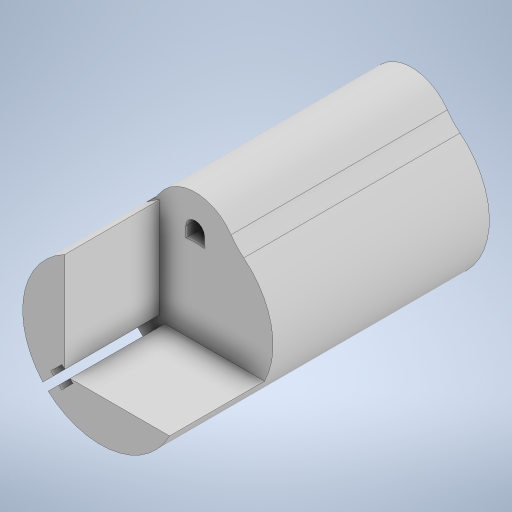
# Autodesk Inventor part: LandingFoot2
Saved by Autodesk Inventor 2023 (Build 270158000, 158)
## iProperties
Created: 2023-01-25
Part Number: LandingFoot2
Material: Generic
Document SubType Name: Modeling
Designer: chase
Density: 1 g/cm^3
Appearance: Default
Author: chase
Autodesk Inventor part; units mm, degrees
ref_plane "YZ Plane" through (0, 0, 0) normal (1, 0, 0) x (0, 1, 0)
ref_plane "XZ Plane" through (0, 0, 0) normal (0, 1, 0) x (-1, 0, 0)
ref_plane "XY Plane" through (0, 0, 0) normal (0, 0, 1) x (1, 0, 0)
sketch "Sketch1" plane through (0, 0, 0) normal (0, 0, 1) x (1, 0, 0)
  circle A0 centre (0, 0) radius 12.5
  dimension "d0" = 25
  constraints: 1 centre point, 1 coincident
  measures "d0" diameter of A0
extrude "Extrusion1" add sketch "Sketch1" against normal blind 50
sketch "Sketch2" plane through (0, 0, -50) normal (0, 0, -1) x (-1, 0, 0)
  circle A0 centre (0, 0) radius 8.075
  dimension "d3" = 16.15
  constraints: 1 centre point, 1 coincident
  measures "d3" diameter of A0
extrude "Extrusion2" cut sketch "Sketch2" against normal blind 25.4
sketch "Sketch3" plane through (0, 0, 0) normal (0, 0, 1) x (1, 0, 0)
  circle A0 centre (0, 0) radius 12.5
  line L0 (0, 12.5) -> (0, 0) construction
  line L1 (0, 0) -> (-8.8388, -8.8388) construction
  line L2 (-4.4194, -2.6517) -> (-9.7227, -7.955)
  line L3 (-9.7227, -7.955) -> (-7.955, -9.7227)
  line L4 (-7.955, -9.7227) -> (-2.6517, -4.4194)
  line L5 (-9.7227, -7.955) -> (-7.955, -9.7227)
  line L6 (-6.1872, -4.4194) -> (-4.4194, -6.1872)
  line L7 (-7.955, -6.1872) -> (-6.1872, -7.955)
  line L8 (-8.4146, -9.2631) -> (-6.6468, -7.4953)
  line L9 (-9.2631, -8.4146) -> (-7.4953, -6.6468)
  line L10 (-4.4194, -2.6517) -> (-2.6517, -4.4194)
  line L11 (-4.879, -5.7276) -> (-4.5255, -5.374)
  line L12 (-5.7276, -4.879) -> (-5.374, -4.5255)
  line L13 (-5.374, -4.5255) -> (-4.5255, -5.374)
  line L14 (-4.9497, -4.9497) -> (-3.5355, -3.5355)
  line L15 (-5.2679, -4.6315) -> (-3.8537, -3.2173)
  line L16 (-4.6315, -5.2679) -> (-3.2173, -3.8537)
  line L17 (-4.4194, -2.6517) -> (-2.6517, -4.4194)
  line L18 (-4.879, -5.7276) -> (11.1106, -5.7276)
  line L19 (-5.7276, -4.879) -> (-5.7276, 11.1106)
  constraints: 40 end point, 6 point on line, 1 vertical, 3 other
extrude "Extrusion3" cut sketch "Sketch3" against normal blind 15.24 contours A0 L18 L4 L10 L2 L19 | L2 L10 L15 L13 L12 L19 | L18 L11 L13 L16 L10 L4 | L9 L7 L8 A0 | A0 L3 L9 | L2 L6 L4 L7 | L12 L13 L11 L6 | L8 L3 A0 | L10 L14 L13 L15 | L16 L13 L14 L10
sketch "Sketch4" plane through (0, 0, -50) normal (0, 0, -1) x (-1, 0, 0)
  arc A0 (6.4283, 10.7204) -> (-6.4283, 10.7204) centre (0, 8.075) ccw
  arc A1 (1.5, 7.9345) -> (-1.5, 7.9345) centre (0, 0) ccw
  circle A2 centre (0, 0) radius 12.5
  point P0 (0, 8.075)
  dimension "d17" = 12.8567
  dimension "d18" = 6.4283
  constraints: 8 point on circle, 3 centre point
  measures "d17" distance of A0.start A0.end
  measures "d18" horizontal distance of A0.start point (0, 8.075)
extrude "Extrusion4" add sketch "Sketch4" against normal up to surface (34.76 mm away) contours A2 A0
sketch "Sketch5" plane through (0, 0, -50) normal (0, 0, -1) x (-1, 0, 0)
  circle A0 centre (0, 9.575) radius 1.5
  line L0 (-1.5, 9.575) -> (-1.5, 7.9345)
  line L1 (1.5, 9.575) -> (1.5, 7.9345)
  circle A1 centre (0, 0) radius 8.075
  dimension "d21" = 3
  dimension "d22" = 16.15
  constraints: 4 end point, 2 centre point, 2 point on circle, 1 coincident, 1 parallel, 1 vertical
  measures "d21" diameter of A0
  measures "d22" diameter of A1
extrude "Extrusion5" cut sketch "Sketch5" against normal up to surface (34.76 mm away) contours A0 | L1 A1 A0 | A0 A1 L0
fillet "Fillet1" radius 10 2 edges at (6.4283, 10.7204, -32.62) (-6.4283, 10.7204, -32.62)
equation "\"d18\" = 0.5 * d17"
body "Solid1"
